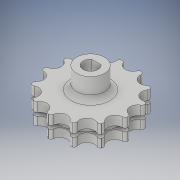
# Autodesk Inventor part: chain_gear
Saved by Autodesk Inventor 2017 (Build 210142000, 142)
## iProperties
Created: 2018-09-27
Part Number: chain_gear
Material: Generic
Document SubType Name: Modeling
Designer: Mitch
Density: 1 g/cm^3
Appearance: Default
Author: Mitch
Autodesk Inventor part; units mm, degrees
ref_plane "YZ Plane" through (0, 0, 0) normal (1, 0, 0) x (0, 1, 0)
ref_plane "XZ Plane" through (0, 0, 0) normal (0, 1, 0) x (-1, 0, 0)
ref_plane "XY Plane" through (0, 0, 0) normal (0, 0, 1) x (1, 0, 0)
sketch "Sketch1" plane through (0, 0, 0) normal (0, 1, 0) x (-1, 0, 0)
  circle A0 centre (0, 0) radius 12.7
  dimension "d0" = 25.4
  constraints: 1 centre point, 1 coincident
  measures "d0" diameter of A0
extrude "Extrusion1" add sketch "Sketch1" along normal blind 6.35
sketch "Sketch2" plane through (0, 6.35, 0) normal (0, 1, 0) x (1, 0, 0)
  circle A0 centre (0, 0) radius 12.7 projected
  circle A1 centre (0, 12.7) radius 2.2606
  circle A2 centre (-5.902, 11.2453) radius 2.2606
  circle A3 centre (-10.4519, 7.2144) radius 2.2606
  circle A4 centre (-12.6074, 1.5308) radius 2.2606
  circle A5 centre (-11.8747, -4.5035) radius 2.2606
  circle A6 centre (-8.4217, -9.5061) radius 2.2606
  circle A7 centre (-3.0393, -12.331) radius 2.2606
  circle A8 centre (3.0393, -12.331) radius 2.2606
  circle A9 centre (8.4217, -9.5061) radius 2.2606
  circle A10 centre (11.8747, -4.5035) radius 2.2606
  circle A11 centre (12.6074, 1.5308) radius 2.2606
  circle A12 centre (10.4519, 7.2144) radius 2.2606
  circle A13 centre (5.902, 11.2453) radius 2.2606
  dimension "d8" = 4.5212
  dimension "d11" = 360
  constraints: 13 centre point, 1 vertical alignment, 28 other
  measures "d8" diameter of A1
sketch "Sketch4" plane through (0, 6.35, 0) normal (0, 1, 0) x (1, 0, 0)
  circle A0 centre (0, 0) radius 4.191
  dimension "d18" = 8.382
  constraints: 1 centre point, 1 coincident
  measures "d18" diameter of A0
extrude "Extrusion3" add sketch "Sketch4" along normal blind 6.35
fillet "Fillet1" radius 1.5875 1 edges at (-4.191, 6.35, 0)
sketch "Sketch5" plane through (0, 12.7, 0) normal (0, 1, 0) x (1, 0, 0)
  arc A0 (-1.3524, 1.4478) -> (1.3524, 1.4478) centre (0, 0) ccw
  line L0 (0, -1.9812) -> (0, 1.4478)
  line L1 (0, 1.4478) -> (1.3524, 1.4478)
  line L2 (0, 1.4478) -> (-1.3524, 1.4478)
  line L3 (1.4491, 1.7018) -> (0, 1.7018)
  line L4 (0, 1.7018) -> (-1.4491, 1.7018)
  arc A1 (-1.4491, 1.7018) -> (1.4491, 1.7018) centre (0, 0) ccw
  dimension "d22" = 3.9624
  dimension "d23" = 3.429
  dimension "d35" = 0.254
  constraints: 10 end point, 5 point on circle, 2 centre point, 2 horizontal, 1 coincident, 1 vertical, 2 other
  measures "d22" diameter of A0
  measures "d23" distance of L0.start L0.end
  measures "d35" distance between parallel lines of L1 L3
ref_plane "Work Plane2" through (0, 2.54, 0) normal (0, 1, 0) x (1, 0, 0)
sketch "Sketch6" plane through (0, 2.54, 0) normal (0, 1, 0) x (1, 0, 0)
  circle A0 centre (0, 0) radius 12.7
  circle A1 centre (0, 0) radius 10.16
  dimension "d28" = 25.4
  dimension "d29" = 2.54
  constraints: 2 centre point, 1 coincident
  measures "d28" diameter of A0
  measures "d29" radial gap between concentric circles of A0 A1
extrude "Extrusion5" cut sketch "Sketch6" along normal blind 1.016
extrude "Extrusion7" cut sketch "Sketch5" against normal blind 25.4 contours L2 L0 A0 | L0 L1 A0 | A1 L4 L3
extrude "Extrusion8" cut sketch "Sketch2" against normal blind 25.4 contours A0 A11 | A0 A11 | A12 A0 | A0 A12 | A10 A0 | A0 A10 | A13 A0 | A0 A13 | A9 A0 | A0 A9 | A1 A0 | A0 A1 | A8 A0 | A0 A8 | A2 A0 | A0 A2 | A7 A0 | A0 A7 | A3 A0 | A0 A3 | A6 A0 | A0 A6 | A4 A0 | A0 A4 | A5 A0 | A0 A5
fillet "Fillet4" radius 0.7937 52 edges at (-5.1774, 1.27, 11.5968) (-5.1774, 4.953, 11.5968) (-6.6029, 1.27, 10.8486) (-6.6029, 4.953, 10.8486) (0.805, 1.27, 12.6745) (0.805, 4.953, 12.6745) (-0.805, 1.27, 12.6745) (-0.805, 4.953, 12.6745) (6.6029, 1.27, 10.8486) (6.6029, 4.953, 10.8486) (5.1774, 1.27, 11.5968) (5.1774, 4.953, 11.5968) (10.8881, 1.27, 6.5374) (10.8881, 4.953, 6.5374) (9.9736, 1.27, 7.8624) (9.9736, 4.953, 7.8624) (12.485, 1.27, 2.3268) (12.485, 4.953, 2.3268) (12.6791, 1.27, 0.7286) (12.6791, 4.953, 0.7286) (12.1363, 1.27, -3.7418) (12.1363, 4.953, -3.7418) (11.5654, 1.27, -5.2471) (11.5654, 4.953, -5.2471) (9.0072, 1.27, -8.9532) (9.0072, 4.953, -8.9532) (7.8022, 1.27, -10.0208) (7.8022, 4.953, -10.0208) (3.8148, 1.27, -12.1135) (3.8148, 4.953, -12.1135) (2.2516, 1.27, -12.4988) (2.2516, 4.953, -12.4988) (-2.2516, 1.27, -12.4988) (-2.2516, 4.953, -12.4988) (-3.8148, 1.27, -12.1135) (-3.8148, 4.953, -12.1135) (-7.8022, 1.27, -10.0208) (-7.8022, 4.953, -10.0208) (-9.0072, 1.27, -8.9532) (-9.0072, 4.953, -8.9532) (-11.5654, 1.27, -5.2471) (-11.5654, 4.953, -5.2471) (-12.1363, 1.27, -3.7418) (-12.1363, 4.953, -3.7418) (-12.6791, 1.27, 0.7286) (-12.6791, 4.953, 0.7286) (-12.485, 1.27, 2.3268) (-12.485, 4.953, 2.3268) (-10.8881, 1.27, 6.5374) (-10.8881, 4.953, 6.5374) (-9.9736, 1.27, 7.8624) (-9.9736, 4.953, 7.8624)
body "Solid1"
